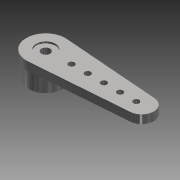
# Autodesk Inventor part: ServoHorn
Saved by Autodesk Inventor 2014 (Build 180170000, 170)
## iProperties
Created: 2014-02-25
Part Number: ServoHorn
Material: Generic
Document SubType Name: Modeling
Designer: Jonathan
Density: 1 g/cm^3
Appearance: Default
Author: Jonathan
Autodesk Inventor part; units mm, degrees
ref_plane "YZ Plane" through (0, 0, 0) normal (1, 0, 0) x (0, 1, 0)
ref_plane "XZ Plane" through (0, 0, 0) normal (0, 1, 0) x (-1, 0, 0)
ref_plane "XY Plane" through (0, 0, 0) normal (0, 0, 1) x (1, 0, 0)
sketch "Sketch1" plane through (0, 0, 0) normal (0, 1, 0) x (-1, 0, 0)
  arc A0 (-0.5058, -6.4803) -> (-0.5058, 6.4803) centre (0, 0) ccw
  arc A1 (-32.3013, 3.9986) -> (-32.3013, -3.9986) centre (-31.9892, 0) ccw
  line L0 (-32.3013, -3.9986) -> (-0.5058, -6.4803)
  line L1 (-0.5058, 6.4803) -> (-32.3013, 3.9986)
  circle A2 centre (0, 0) radius 1.47
  circle A3 centre (-14, 0) radius 1
  circle A4 centre (-19.4, 0) radius 1
  circle A5 centre (-24.8, 0) radius 1
  circle A6 centre (-30.2, 0) radius 1
  circle A7 centre (-8.6, 0) radius 1
  point P0 (-36, 0)
  point P1 (-36, 0)
  dimension "d0" = 0
  dimension "d1" = 0
  dimension "d2" = 13
  dimension "d3" = 0
  dimension "d4" = 42.5
  dimension "d5" = 2.94
  dimension "d6" = 5.4
  dimension "d7" = 5.4
  dimension "d8" = 5.4
  dimension "d9" = 5.4
  dimension "d10" = 0
  dimension "d11" = 5.8
  dimension "d12" = 2
  dimension "d13" = 2
  dimension "d14" = 2
  dimension "d15" = 2
  dimension "d16" = 2
  dimension "d17" = 0
  dimension "d18" = 0
  dimension "d19" = 0
  dimension "d20" = 0
  dimension "d21" = 0
  dimension "d22" = 3.15
  constraints: 8 centre point, 5 point on circle, 4 end point, 4 tangent, 2 coincident
  measures "d0" distance of point (0, 0) A0.centre
  measures "d1" distance of point (0, 0) A0.centre
  measures "d2" diameter of A0
  measures "d3" vertical distance of A1.centre point (0, 0)
  measures "d5" diameter of A2
  measures "d6" distance of A5.centre A4.centre
  measures "d7" distance of A3.centre A4.centre
  measures "d8" distance of A7.centre A3.centre
  measures "d9" distance of A6.centre A5.centre
  measures "d10" vertical distance of A6.centre A1.centre
  measures "d11" distance of A6.centre point (-36, 0)
  measures "d12" diameter of A6
  measures "d13" diameter of A5
  measures "d14" diameter of A4
  measures "d15" diameter of A3
  measures "d16" diameter of A7
  measures "d17" vertical distance of A3.centre A7.centre
  measures "d18" vertical distance of A4.centre A3.centre
  measures "d19" vertical distance of A5.centre A4.centre
  measures "d20" vertical distance of A6.centre A5.centre
  measures "d21" vertical distance of point (0, 0) point (-36, 0)
  measures "d22" distance edge to line of A6 L0
extrude "Extrusion1" add sketch "Sketch1" along normal blind 2.8
sketch "Sketch2" plane through (0, 0, 0) normal (0, -1, 0) x (1, 0, 0)
  circle A0 centre (0, 0) radius 3.365 construction
  arc A1 (0.5058, 6.4803) -> (0.5058, -6.4803) centre (0, 0) ccw projected
  circle A2 centre (0, 0) radius 5.515
  circle A3 centre (0, 0) radius 3.365
  dimension "d25" = 11.03
  dimension "d28" = 6.73
  constraints: 3 centre point, 2 coincident, 1 concentric
  measures "d25" diameter of A2
  measures "d28" diameter of A0
extrude "Extrusion3" add sketch "Sketch2" along normal blind 6
sketch "Sketch3" plane through (0, 2.8, 0) normal (0, 1, 0) x (1, 0, 0)
  circle A0 centre (0, 0) radius 1.47 projected
  arc A1 (0.5058, 6.4803) -> (0.5058, -6.4803) centre (0, 0) ccw projected
  circle A2 centre (0, 0) radius 3.2
  dimension "d31" = 6.4
  constraints: 1 centre point, 1 coincident
  measures "d31" diameter of A2
extrude "Extrusion4" cut sketch "Sketch3" against normal blind 0.56
equation "\"d7\" = d6"
equation "\"d8\" = d6"
equation "\"d9\" = d6"
equation "\"d13\" = d12"
equation "\"d14\" = d12"
equation "\"d15\" = d12"
equation "\"d16\" = d12"
body "Solid1"
